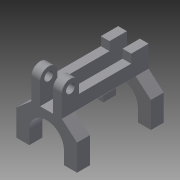
# Autodesk Inventor part: 3-4
Saved by Autodesk Inventor 2015 SP2 (Build 190223200, 223)
## iProperties
Created: 2015-09-14
Part Number: 3-4
Material: Generic
Document SubType Name: Modeling
Designer: Brandon
Density: 1 g/cm^3
Appearance: Default
Author: Brandon
Autodesk Inventor part; units mm, degrees
ref_plane "YZ Plane" through (0, 0, 0) normal (1, 0, 0) x (0, 1, 0)
ref_plane "XZ Plane" through (0, 0, 0) normal (0, 1, 0) x (-1, 0, 0)
ref_plane "XY Plane" through (0, 0, 0) normal (0, 0, 1) x (1, 0, 0)
sketch "Sketch1" plane through (0, 0, 0) normal (0, 0, 1) x (1, 0, 0)
  line L0 (0, 0) -> (88.9, 0)
  line L1 (22.225, 57.15) -> (22.225, 88.9)
  line L2 (22.225, 88.9) -> (66.675, 88.9)
  line L3 (66.675, 88.9) -> (66.675, 57.15)
  line L4 (88.9, 0) -> (88.9, 38.1)
  line L5 (88.9, 38.1) -> (66.675, 57.15)
  line L6 (0, 0) -> (0, 38.1)
  line L7 (0, 38.1) -> (22.225, 57.15)
  line L8 (22.225, 57.15) -> (66.675, 57.15)
  dimension "d4" = 44.45
  dimension "d12" = 38.1
  dimension "d13" = 38.1
  dimension "d14" = 44.45
  dimension "d15" = 31.75
  dimension "d16" = 88.9
  constraints: 18 end point, 2 horizontal, 1 perpendicular
  measures "d4" distance of L1.end L2.end
  measures "d12" distance of L0.end L4.end
  measures "d13" distance of L0.start L6.end
  measures "d14" distance of L1.start L3.end
  measures "d15" distance of L1.start L1.end
  measures "d16" distance of L0.start L0.end
extrude "Extrusion1" add sketch "Sketch1" along normal blind 127
sketch "Sketch2" plane through (0, 0, 127) normal (0, 0, 1) x (1, 0, 0)
  line L0 (0, 0) -> (88.9, 0) projected
  line L1 (44.45, 0) -> (44.45, 19.05)
  circle A0 centre (44.45, 19.05) radius 25.4
  line L2 (19.05, 19.05) -> (19.05, 0)
  line L3 (69.85, 0) -> (69.85, 19.05)
  dimension "d8" = 19.05
  dimension "d9" = 50.8
  constraints: 6 end point, 2 point on circle, 2 point on line, 1 centre point, 1 coincident, 1 midpoint, 1 perpendicular, 1 tangent, 1 vertical
  measures "d8" distance of L1.start L1.end
  measures "d9" diameter of A0
extrude "Extrusion2" cut sketch "Sketch2" against normal through all
sketch "Sketch3" plane through (0, 0, 127) normal (0, 0, 1) x (1, 0, 0)
  line L0 (22.225, 88.9) -> (34.925, 88.9)
  line L1 (66.675, 88.9) -> (22.225, 88.9) projected
  line L2 (34.925, 88.9) -> (53.975, 88.9)
  line L3 (53.975, 88.9) -> (66.675, 88.9)
  line L4 (34.925, 88.9) -> (34.925, 57.15)
  line L5 (53.975, 88.9) -> (53.975, 57.15)
  line L6 (53.975, 57.15) -> (34.925, 57.15)
  point P0 (0, 0)
  point P1 (22.225, 57.15)
  point P2 (66.675, 57.15)
  dimension "d17" = 12.7
  dimension "d18" = 19.05
  constraints: 12 end point, 2 point on line, 1 collinear, 1 perpendicular, 1 vertical
  measures "d17" distance of L0.start L0.end
  measures "d18" distance of L0.end L2.end
extrude "Extrusion3" cut sketch "Sketch3" against normal through all
sketch "Sketch4" plane through (88.9, 0, 0) normal (1, 0, 0) x (0, 0, -1)
  line L0 (-127, 0) -> (-107.95, 0)
  line L1 (0, 0) -> (-127, 0) projected
  line L2 (-107.95, 0) -> (-107.95, 56.6372)
  line L3 (-107.95, 56.6372) -> (-19.0515, 57.15)
  line L4 (0, 57.15) -> (-127, 57.15) projected
  line L5 (-19.0515, 57.15) -> (-18.7218, 0)
  dimension "d21" = 19.05
  dimension "d22" = 88.9
  constraints: 8 end point, 3 point on line, 2 perpendicular
  measures "d21" distance of L0.start L0.end
  measures "d22" distance of L2.end L3.end
extrude "Extrusion4" cut sketch "Sketch4" against normal through all
sketch "Sketch5" plane through (66.675, 57.15, 0) normal (1, 0, 0) x (0, 0, -1)
  line L0 (0, 31.75) -> (-25.4, 31.75)
  line L1 (0, 31.75) -> (-127, 31.75) projected
  line L2 (-25.4, 31.75) -> (-25.4, 19.05)
  line L3 (-25.4, 19.05) -> (-101.6, 19.05)
  line L4 (-101.6, 19.05) -> (-101.6, 31.75)
  point P0 (0, -57.15)
  dimension "d25" = 25.4
  dimension "d26" = 12.7
  dimension "d27" = 76.2
  constraints: 8 end point, 3 perpendicular, 2 point on line
  measures "d25" distance of L0.start L0.end
  measures "d26" distance of L0.end L2.end
  measures "d27" distance of L2.end L3.end
extrude "Extrusion5" cut sketch "Sketch5" against normal through all
sketch "Sketch6" plane through (66.675, 57.15, 0) normal (1, 0, 0) x (0, 0, -1)
  line L0 (-101.6, 31.75) -> (-127, 31.75) projected
  circle A0 centre (-114.3, 31.75) radius 12.7
  point P0 (0, -57.15)
  constraints: 1 horizontal alignment, 1 midpoint, 2 other
extrude "Extrusion6" add sketch "Sketch6" against normal blind 44.45
sketch "Sketch7" plane through (0, 0, 127) normal (0, 0, 1) x (1, 0, 0)
  line L0 (66.675, 101.6) -> (22.225, 101.6) projected
  line L1 (34.925, 57.15) -> (53.975, 57.15)
  line L2 (53.975, 57.15) -> (53.975, 101.6)
  line L3 (53.975, 101.6) -> (34.925, 101.6)
  line L4 (34.925, 101.6) -> (34.925, 57.15)
  point P0 (0, 0)
  constraints: 8 end point, 2 parallel, 1 horizontal, 1 perpendicular, 1 point on line
extrude "Extrusion7" cut sketch "Sketch7" against normal blind 44.45
sketch "Sketch8" plane through (66.675, 57.15, 0) normal (1, 0, 0) x (0, 0, -1)
  line L0 (-127, 31.75) -> (-101.7646, 31.75)
  circle A0 centre (-114.3823, 31.75) radius 6.35
  point P0 (0, -57.15)
  dimension "d34" = 12.7
  constraints: 2 end point, 1 centre point, 1 horizontal, 1 midpoint
  measures "d34" diameter of A0
extrude "Extrusion8" cut sketch "Sketch8" against normal through all
body "Solid1"
